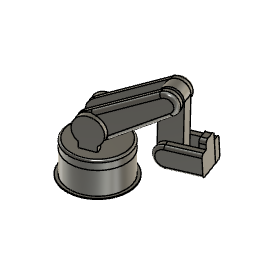
Garra pet v5 (Autodesk Fusion 360 design; units mm, degrees)
Autodesk Fusion 360 part; units mm, degrees
sketch "Esboço1" plane through (0, 0, 0) normal (0, 0, 1) x (1, 0, 0) in component "Component"
  circle A0 centre (0, 0) radius 82.5
  dimension "d1" = 165
  constraint coincident A0.centre origin
  measures "d1" diameter of A0
extrude "Extrusão1" add sketch "Esboço1" along normal blind 2 makes body 1 in component "Component"
ref_plane "Plano de trabalho1" through (0, 0, 2) normal (0, 0, 1) x (1, 0, 0) in component "Component"
sketch "Esboço2" plane through (0, 0, 2) normal (0, 0, 1) x (1, 0, 0) in component "Component"
  circle A0 centre (0, 0) radius 75
  dimension "d5" = 150
  constraint coincident A0.centre origin
  measures "d5" diameter of A0
extrude "Extrusão2" add sketch "Esboço2" along normal blind 60 bodies 1 in component "Component"
ref_plane "Plano de trabalho2" through (0, 0, 67) normal (0, 0, 1) x (1, 0, 0) in component "Component"
sketch "Esboço3" plane through (0, 0, 67) normal (0, 0, 1) x (1, 0, 0) in component "Component"
  circle A0 centre (0, 0) radius 40 construction
  circle A1 centre (0, 40) radius 15 construction
  dimension "d9" = 80
  dimension "d10" = 30
  constraint coincident A0.centre origin
  constraint coincident A0 A1.centre
  measures "d9" diameter of A0
  measures "d10" diameter of A1
ref_plane "Plano de trabalho1" through (0, 0, 67) normal (0, 0, 1) x (1, 0, 0) in component "Component'"
sketch "Esboço1 (2)" plane through (0, 0, 67) normal (0, 0, 1) x (1, 0, 0) in component "Component'"
  circle A0 centre (0, 0) radius 75
  dimension "d12" = 150
  constraint coincident A0.centre origin
  measures "d12" diameter of A0
extrude "Extrusão1'" add sketch "Esboço1 (2)" along normal blind 22.6 separate body makes body 2 in component "Component'"
sketch "Esboço2 (2)" plane through (0, 0, 89.6) normal (0, 0, 1) x (-1, 0, 0) in component "Component'"
  circle A0 centre (0, 0) radius 75
  line L0 (0, 0) -> (30, 0) construction
  line L1 (30, 0) -> (0, 0) construction
  line L2 (0, 0) -> (-30, 0) construction
  line L3 (30, 0) -> (30, 20) construction
  line L4 (30, 20) -> (44.6, 20) construction
  line L5 (44.6, 20) -> (44.6, 0) construction
  line L6 (30, 0) -> (30, -20) construction
  line L7 (30, -20) -> (44.6, -20) construction
  line L8 (44.6, -20) -> (44.6, 0) construction
  line L9 (0, 50) -> (0, -45) construction
  line L10 (-30, 0) -> (-30, 20) construction
  line L11 (-30, 0) -> (-30, -20) construction
  line L12 (-30, -20) -> (-44.6, -20) construction
  line L13 (-44.6, -20) -> (-44.6, 0) construction
  line L14 (-44.6, 20) -> (-44.6, 0) construction
  line L15 (-30, 20) -> (-44.6, 20) construction
  dimension "d15" = 30
  dimension "d16" = 30
  dimension "d17" = 20
  dimension "d18" = 14.6
  constraint coincident A0.centre L0.start
  constraint horizontal L0
  constraint parallel L1 L2
  constraint perpendicular L3 L4
  constraint parallel L3 L5
  constraint perpendicular L0 L3
  constraint perpendicular L6 L7
  constraint parallel L6 L8
  constraint perpendicular L0 L6
  constraint perpendicular L0 L9
  constraint symmetric L0.end L9 L2.end
  constraint symmetric L3.end L9 L10.end
  constraint symmetric L4.end L9 L14.start
  constraint symmetric L5.end L9 L13.end
  constraint symmetric L6.end L9 L11.end
  constraint symmetric L7.end L9 L12.end
  measures "d15" distance of A0.centre L0.end
  measures "d16" distance of A0.centre L2.end
  measures "d17" distance of L0.end L3.end
  measures "d18" distance of L0.end L5.end
ref_plane "Plano de trabalho2" through (0, -50, 89.6) normal (-1, 0, 0) x (0, -1, 0) in component "Component'"
ref_plane "Plano de trabalho3" through (-30, -50, 89.6) normal (-1, 0, 0) x (0, -1, 0) in component "Component'"
sketch "Esboço3 (2)" plane through (-30, 0, 0) normal (-1, 0, 0) x (0, -1, 0) in component "Component'"
  line L0 (0, 90) -> (0, 133) construction
  circle A0 centre (0, 133) radius 35
  line L1 (-20, 90) -> (-20, 104.2772)
  line L2 (20, 90) -> (20, 104.2772)
  line L3 (20, 90) -> (-20, 90)
  dimension "d20" = 43
  dimension "d21" = 70
  constraint vertical L0
  constraint coincident L0.end A0.centre
  constraint coincident A0 L1.end
  constraint parallel L0 L1
  constraint coincident A0 L2.end
  constraint parallel L0 L2
  constraint perpendicular L1 L3
  measures "d20" distance of L0.start L0.end
  measures "d21" diameter of A0
extrude "Extrusão2'" add sketch "Esboço3 (2)" along normal blind 14.6 separate body makes body 3 in component "Component'"
mirror "Espelhar1" about plane through (0, -50, 89.6) normal (-1, 0, 0) of bodies 3 makes body 4 in component "Component'"
ref_plane "Plano de trabalho1" through (0, 0, 129) normal (1, 0, 0) x (0, 1, 0) in component "Component''"
ref_plane "Plano de trabalho2" through (18.375, 0, 129) normal (1, 0, 0) x (0, 1, 0) in component "Component''"
sketch "Esboço1 (3)" plane through (18.375, 0, 0) normal (1, 0, 0) x (0, 1, 0) in component "Component''"
  line L0 (0, 90) -> (0, 133) construction
  line L1 (0, 133) -> (187.5, 133) construction
  line L2 (0, 133) -> (0, 168) construction
  line L3 (187.5, 133) -> (187.5, 160.5) construction
  line L4 (0, 133) -> (0, 98) construction
  line L5 (187.5, 133) -> (187.5, 105.5) construction
  line L6 (0, 168) -> (187.5, 160.5)
  line L7 (0, 98) -> (187.5, 105.5)
  arc A0 (2.7955, 167.8882) -> (2.7955, 98.1118) centre (0, 133) ccw
  arc A1 (187.5, 105.5) -> (187.5, 160.5) centre (187.5, 133) ccw
  dimension "d27" = 43
  dimension "d28" = 70
  dimension "d29" = 187.5
  dimension "d30" = 55
  constraint vertical L0
  constraint coincident L0.end L1.start
  constraint perpendicular L0 L1
  constraint coincident L1.end L3.start
  constraint coincident L2.end A0
  constraint vertical L2
  constraint perpendicular L1 L3
  constraint coincident L4.end A0
  constraint coincident L0 L4.end
  constraint parallel L0 L5
  constraint coincident L6 A0.start
  constraint coincident L7 A0.end
  measures "d27" distance of L0.start L0.end
  measures "d28" diameter of A0
  measures "d29" distance of L0.end L1.end
  measures "d30" diameter of A1
extrude "Extrusão1''" add sketch "Esboço1 (3)" along normal blind 9.6 separate body contours L6 L7 A0 A1 makes body 5 in component "Component''"
ref_plane "Plano de trabalho3" through (27.975, 90, 133) normal (1, 0, 0) x (0, 1, 0) in component "Component''"
sketch "Esboço2 (3)" plane through (27.975, 0, 0) normal (1, 0, 0) x (0, 1, 0) in component "Component''"
  arc A0 (0, 168) -> (0, 98) centre (0, 133) ccw
  line L0 (0, 98) -> (187.5, 105.5)
  arc A1 (187.5, 105.5) -> (187.5, 160.5) centre (187.5, 133) ccw
  line L1 (187.5, 160.5) -> (0, 168)
  arc A2 (20, 104.2772) -> (-20, 104.2772) centre (0, 133) ccw construction
  line L2 (-20, 104.2772) -> (-20, 90) construction
  line L3 (-20, 90) -> (20, 90) construction
  line L4 (20, 90) -> (20, 104.2772) construction
  line L5 (22.5, 98.9) -> (22.5, 103) construction
  line L6 (0, 133) -> (187.5, 133) construction
  line L7 (22.5, 167.1) -> (22.5, 163) construction
  line L8 (22.5, 163) -> (22.5, 167.1)
  line L9 (22.5, 167.1) -> (187.5, 160.5)
  line L10 (22.5, 98.9) -> (187.5, 105.5)
  arc A3 (22.5, 103) -> (22.5, 163) centre (0, 133) ccw
  arc A4 (22.5, 103) -> (-20, 101.2786) centre (0, 133) ccw construction
  line L11 (22.5, 103) -> (22.5, 98.9)
  arc A5 (187.5, 105.5) -> (187.5, 160.5) centre (187.5, 133) ccw
  dimension "d34" = 75
  constraint concentric A0 A4
  constraint parallel L4 L5
  constraint coincident A0.centre A2.centre
  constraint coincident A1.centre L6.end
  constraint symmetric L5.end L6 L7.end
  constraint concentric A1 A5
  constraint concentric A0 A3
  constraint coincident L1 L7.start
  constraint coincident A1.end L1.start
  constraint symmetric L6 L7.start L5.start
  constraint symmetric L6 A1.end L0.end
  constraint coincident L2 A4.end
  measures "d34" diameter of A4
extrude "Extrusão2''" add sketch "Esboço2 (3)" along normal blind 10 contours L0 A1 L1 L8 L9 L10 A3 L11 A5 bodies 5 in component "Component''"
mirror "Espelhar1'" about plane through (0, 0, 129) normal (1, 0, 0) of "Extrusão1''", "Extrusão2''" makes body 6 in component "Component''"
ref_plane "Plano de trabalho1" through (-18.375, 90, 133) normal (1, 0, 0) x (0, -1, 0)
sketch "Esboço1 (4)" plane through (-18.375, 0, 0) normal (1, 0, 0) x (0, 1, 0)
  arc A0 (20, 104.2772) -> (-20, 104.2772) centre (0, 133) ccw
  line L0 (-20, 104.2772) -> (-20, 90)
  line L1 (-20, 90) -> (20, 90)
  line L2 (20, 90) -> (20, 104.2772)
  line L3 (22.5, 103) -> (22.5, 98.9)
  line L4 (22.5, 98.9) -> (187.5, 105.5)
  arc A1 (187.5, 105.5) -> (187.5, 160.5) centre (187.5, 133) ccw
  line L5 (187.5, 160.5) -> (22.5, 167.1)
  line L6 (22.5, 167.1) -> (22.5, 163)
  arc A2 (22.5, 103) -> (22.5, 163) centre (0, 133) ccw
  line L7 (0, 133) -> (187.5, 133) construction
  circle A3 centre (126.25, 133) radius 5
  circle A4 centre (61.25, 133) radius 5
  point P0 (61.25, 133)
  point P1 (126.25, 133)
  point P2 (93.75, 133)
  dimension "d41" = 65
  dimension "d42" = 93.75
  dimension "d43" = 32.5
  dimension "d44" = 10
  dimension "d45" = 10
  constraint coincident A0.centre A2.centre
  constraint coincident A1.centre L7.end
  constraint coincident L7 P0
  constraint coincident L7 P1
  constraint coincident L7 P2
  constraint coincident P1 A3.centre
  constraint coincident P0 A4.centre
  measures "d41" distance of P0 P1
  measures "d42" distance of A1.centre P2
  measures "d43" distance of P1 P2
  measures "d44" diameter of A3
  measures "d45" diameter of A4
extrude "Extrusão3" add sketch "Esboço1 (4)" along normal blind 40 contours A3 | A4 bodies 5 6 in component "Component''"
ref_plane "Plano de trabalho1" through (0, 90, 133) normal (1, 0, 0) x (0, -1, 0) in component "Component'''"
ref_plane "Plano de trabalho2" through (-15, 90, 133) normal (1, 0, 0) x (0, -1, 0) in component "Component'''"
sketch "Esboço1 (5)" plane through (-15, 0, 0) normal (1, 0, 0) x (0, 1, 0) in component "Component'''"
  line L0 (22.5, 103) -> (22.5, 98.9)
  line L1 (22.5, 98.9) -> (187.5, 105.5)
  arc A0 (187.5, 105.5) -> (187.5, 160.5) centre (187.5, 133) ccw
  line L2 (187.5, 160.5) -> (22.5, 167.1)
  line L3 (22.5, 167.1) -> (22.5, 163)
  arc A1 (22.5, 103) -> (22.5, 163) centre (0, 133) ccw
  circle A2 centre (126.25, 133) radius 5
  circle A3 centre (61.25, 133) radius 5
  arc A4 (0, 168) -> (0, 98) centre (0, 133) ccw
  line L4 (0, 98) -> (187.5, 105.5)
  arc A5 (187.5, 105.5) -> (187.5, 160.5) centre (187.5, 133) ccw
  line L5 (187.5, 160.5) -> (0, 168)
  line L6 (126.25, 133) -> (175.332, 108.5617) construction
  line L7 (187.5, 133) -> (77.841, 187.6) construction
  line L8 (126.25, 133) -> (65.673, 163.1617) construction
  line L9 (90.009, 212.0383) -> (199.668, 157.4383)
  line L10 (120.4314, 135.8971) -> (65.673, 163.1617)
  line L11 (132.0686, 130.1029) -> (175.332, 108.5617)
  arc A6 (132.0686, 130.1029) -> (120.4314, 135.8971) centre (126.25, 133) ccw construction
  arc A7 (132.0686, 130.1029) -> (120.4314, 135.8971) centre (126.25, 133) ccw
  arc A8 (90.009, 212.0383) -> (65.673, 163.1617) centre (77.841, 187.6) ccw
  arc A9 (175.332, 108.5617) -> (199.668, 157.4383) centre (187.5, 133) ccw
  dimension "d49" = 54.6
  dimension "d50" = 13
  dimension "d51" = 122.5
  dimension "d52" = 54.6
  constraint concentric A5 A9
  constraint concentric A2 A6
  constraint coincident A2.centre L6.start
  constraint tangent L6 A9
  constraint coincident A0.centre A5.centre
  constraint parallel L6 L7
  constraint coincident L7.end A8.centre
  constraint tangent L8 A8
  constraint tangent L9 A8
  constraint tangent L9 A9
  constraint coincident L8 L10.start
  constraint coincident L6 L11.start
  constraint coincident L10.start A6.end
  constraint parallel L8 L10
  constraint coincident L11.start A6.start
  measures "d49" diameter of A9
  measures "d50" diameter of A6
  measures "d51" distance of A0.centre L7.end
  measures "d52" diameter of A8
extrude "Extrusão1'''" add sketch "Esboço1 (5)" along normal blind 30 separate body contours A0 L2 A5 L5 L9 L10 L11 A7 A8 A9 | A0 L2 A5 L5 L9 A8 makes body 7 in component "Component'''"
sketch "Esboço1 (6)" plane through (-9.5987, -0.156, 0) normal (-0.999868, -0.016249, 0) x (0.016249, -0.999868, 0) in component "Component''''"
  line L0 (160.2004, 128.1461) -> (159.942, 79.8173)
  arc A0 (159.8725, 66.8175) -> (159.942, 79.8173) centre (159.9073, 73.3174) ccw
  line L1 (159.8725, 66.8175) -> (159.5455, 5.6479)
  arc A1 (159.5455, 5.6479) -> (214.1447, 5.356) centre (186.8451, 5.5019) ccw
  line L2 (214.1447, 5.356) -> (214.7996, 127.8542)
  arc A2 (214.7996, 127.8542) -> (160.2004, 128.1461) centre (187.5, 128.0002) ccw
  line L3 (186.8451, 32.8019) -> (266.8451, 32.8019)
  line L4 (266.8451, 32.8019) -> (266.8451, -21.7977)
  line L5 (266.8451, -21.7977) -> (186.6992, -21.7977)
  arc A3 (186.8451, 32.8019) -> (186.9911, -21.7977) centre (186.8451, 5.5019) ccw
  point P0 (186.6992, -21.7977)
  dimension "d71" = 80
  constraint concentric A1 A3
  constraint midpoint A1 P0
  constraint coincident L3.start A3.start
  constraint tangent L3 A3
  constraint horizontal L3
  constraint perpendicular L3 L4
  constraint coincident P0 L5.end
  constraint perpendicular L4 L5
  constraint coincident L5 A3.end
  measures "d71" distance of L3.start L3.end
extrude "Extrusão1''''" add sketch "Esboço1 (6)" along normal blind 20 separate body contours A1 L2 L3 L4 L5 | A1 L2 L3 L5 A3 makes body 8 in component "Component''''"
ref_plane "Plano de trabalho1" through (8.4407, -187.0601, 66.7511) normal (0.999868, 0.016249, 0) x (0.00732, -0.450434, 0.89278) in component "Component''''"
mirror "Espelhar1''" about plane through (8.4407, -187.0601, 66.7511) normal (0.999868, 0.016249, 0) of bodies 8 makes body 9 in component "Component''''"
move_body "Mover1" bodies 9 to x (1, 0, 0) y (0, 1, 0) z (0, 0, 1) at (3.4, 0, 0) in component "Component''''"
move_body "Mover2" bodies 9 to x (1, 0, 0) y (0, 1, 0) z (0, 0, 1) at (3.4, 0, 0) in component "Component''''"
sketch "Esboço2 (4)" plane through (4.336, -266.8099, 0) normal (0.016249, -0.999868, 0) x (0.999868, 0.016249, 0) in component "Component''''"
  line L0 (-9.6, -21.7977) -> (-9.6, 32.8019)
  line L1 (-9.6, 32.8019) -> (-29.6, 32.8019)
  line L2 (-29.6, 32.8019) -> (-29.6, -21.7977)
  line L3 (-29.6, -21.7977) -> (-9.6, -21.7977)
  line L4 (27.1991, 32.8019) -> (27.1991, -21.7977)
  line L5 (27.1991, -21.7977) -> (47.1991, -21.7977)
  line L6 (47.1991, -21.7977) -> (47.1991, 32.8019)
  line L7 (47.1991, 32.8019) -> (27.1991, 32.8019)
  line L8 (-9.6, -21.7977) -> (27.2, -21.7977)
  line L9 (27.2, -21.7977) -> (27.2, 53.2023)
  line L10 (27.2, 53.2023) -> (-9.6, 53.2023)
  line L11 (-9.6, 53.2023) -> (-9.6, -21.7977)
  dimension "d76" = 36.8
  dimension "d77" = 75
  constraint horizontal L8
  constraint vertical L9
  constraint horizontal L10
  constraint vertical L11
  constraint coincident L0.start L3.end
  measures "d76" distance of L0.start L8.end
  measures "d77" distance of L0.start L10.end
extrude "Extrusão2'''" add sketch "Esboço2 (4)" against normal blind 15 contours L0 L4 L8 L9 L10 L11 bodies 8 9 in component "Component''''"
fillet "Arredondamento1" radius 9 2 edges at (31.4105, -258.8689, 53.2023) (-5.3846, -259.4669, 53.2023) on bodies 8 in component "Component''''"
fillet "Arredondamento2" radius 7.5 6 edges at (50.8795, -226.0857, -21.7977) (-25.9112, -227.2232, -21.7977) (-25.9101, -227.2961, 32.8019) (-27.0036, -160.0051, 5.5749) (50.8807, -226.1587, 32.8019) (49.7871, -158.8677, 5.5749) on bodies 8 in component "Component''''"
fillet "Arredondamento1'" radius 10 6 edges at (-37.975, 105, 102.2) (-37.975, 215, 133) (-37.975, 105, 163.8) (37.975, 215, 133) (37.975, 105, 102.2) (37.975, 105, 163.8) on bodies 5 in component "Component''"
fillet "Arredondamento1''" radius 5 1 edges at (-69.9246, -27.1212, 89.6) on bodies 2 in component "Component'"
component "Component" placed x (1, 0, 0) y (0, 1, 0) z (0, 0, 1) at (0, 0, 0)
component "Component'" placed x (-0.348053, 0.937475, 0) y (-0.937475, -0.348053, 0) z (0, 0, 1) at (0, 0, -5)
component "Component''" placed x (-0.348053, 0.937475, 0) y (0.791177, 0.293737, 0.53643) z (0.502889, 0.186706, -0.843945) at (-67.5891, -22.9335, 240.2447)
component "Component''''" placed x (-0.332787, 0.943002, 0.000692) y (-0.942156, -0.332458, -0.042584) z (-0.039926, -0.014823, 0.999093) at (-26.36, -17.0391, 92.6435)
component "Component'''" placed x (-0.348053, 0.937475, 0) y (0.433735, 0.161031, 0.886534) z (0.831104, 0.308561, -0.462663) at (-45.3958, -11.0938, 123.8896)
